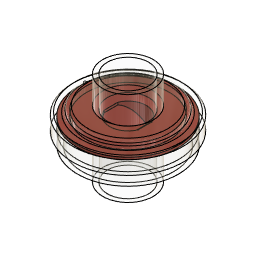
Patient Manifold v2 (Autodesk Fusion 360 design; units mm, degrees)
Autodesk Fusion 360 part; units mm, degrees
sketch "Sketch1" plane through (0, 0, 0) normal (0, 1, 0) x (1, 0, 0)
  line L0 (-20, 0) -> (-20, -10)
  line L1 (-20, -10) -> (-22, -10)
  line L2 (-22, -10) -> (-22, 0)
  line L3 (-22, 0) -> (-20, 0)
  line L4 (-11, -10.0136) -> (-11, 13.9248)
  line L5 (-11, 13.9248) -> (-9, 13.9248)
  line L6 (-9, 13.9248) -> (-9, -10.0136)
  line L7 (-9, -10.0136) -> (-11, -10.0136)
  line L8 (-20, -10) -> (-11, -10.0136)
  line L9 (-20, -8.4865) -> (-11, -8.4865)
  line L10 (-22, -5.5) -> (-24, -5.5)
  line L11 (-24, -5.5) -> (-24, -11.4635)
  line L12 (-23, -12.4635) -> (-20.5, -12.4635)
  line L13 (-22, -10) -> (-22, -11)
  line L14 (-22, -11) -> (-18, -11)
  line L15 (-18, -11) -> (-18, -13.5)
  line L16 (-18, -11) -> (0, -11)
  line L17 (0, -11) -> (0, -2.5)
  line L18 (0, -2.5) -> (-9, -10.0136)
  line L19 (-8.5, -11) -> (0, -4)
  line L20 (-18, -13.5) -> (-9, -13.5)
  line L21 (-9, -13.5) -> (-9, -26.8687)
  line L22 (-9, -26.8687) -> (-11, -26.8687)
  line L23 (-11, -26.8687) -> (-11, -15)
  line L24 (-11, -15) -> (-17.5, -15)
  line L25 (-9, -10.0136) -> (-9, -11)
  line L26 (0, -2.5) -> (-9, -2.5)
  arc A0 (-24, -11.4635) -> (-23, -12.4635) centre (-23, -11.4635) ccw
  arc A1 (-19.5, -13.4635) -> (-20.5, -12.4635) centre (-20.5, -13.4635) ccw
  spline S0 degree 5 poles (-19.5, -13.4635) (-19.5, -13.634) (-19.4835, -13.9431) (-19.4093, -14.312) (-19.2195, -14.6402) (-18.8414, -14.8679) (-18.4111, -14.9593) (-17.9961, -14.9926) (-17.6731, -15) (-17.5, -15) knots 0 0 0 0 0 0 0.2 0.4 0.6 0.8 1 1 1 1 1 1
  line L27 (-17.9, -15) -> (-17.1, -15)
  line L28 (-19.5, -13.1) -> (-19.5, -13.8271)
  dimension "d1" = 2
  dimension "d2" = 2
  dimension "d3" = 11
  dimension "d4" = 20
  dimension "d5" = 9
  dimension "d6" = 11
  dimension "d14" = 1
  constraint vertical L0
  constraint perpendicular L0 L1
  constraint perpendicular L1 L2
  constraint perpendicular L2 L3
  constraint perpendicular L3 L4
  constraint perpendicular L4 L5
  constraint perpendicular L5 L6
  constraint perpendicular L4 L7
  constraint coincident L0 L9.start
  constraint coincident L4 L9.end
  constraint perpendicular L4 L9
  constraint horizontal L10
  constraint perpendicular L10 L11
  constraint perpendicular L11 L12
  constraint perpendicular L1 L13
  constraint perpendicular L13 L14
  constraint perpendicular L14 L15
  constraint perpendicular L15 L16
  constraint perpendicular L14 L17
  constraint coincident L16 L19.start
  constraint coincident L17 L19.end
  constraint perpendicular L15 L20
  constraint perpendicular L20 L21
  constraint perpendicular L21 L22
  constraint perpendicular L20 L23
  constraint perpendicular L21 L24
  constraint midpoint L16 L25.end
  constraint coincident L6 L26.end
  constraint perpendicular L6 L26
  constraint tangent L12 A0
  constraint tangent L11 A0
  constraint tangent L12 A1
  constraint equal A0 A1
  constraint midpoint L24.end L27
  constraint coincident L24 L27.end
  constraint midpoint A1.start L28
  constraint tangent A1 L28
  measures "d1" distance of L4 L6
  measures "d2" distance of L0 L2 L3.end
  measures "d3" distance of origin L4
  measures "d4" distance of origin L0
  measures "d5" distance of L21 origin
  measures "d6" distance of L23 origin
  measures "d14" radius of A0
revolve "Revolve1" add sketch "Sketch1" angle 360 about axis through (0, 0, 1.75) along (0, 0, 1) contours L6 L18 L26 | L16 L17 L18 L19 L25 | L16 L17 L19 makes body 1
extrude "Extrude1" cut sketch "Sketch1" along normal through all and the other way through all contours L6 L18 L26 bodies 1
mirror "Mirror1" about plane through (0, 0, 0) normal (1, 0, 0) of "Extrude1"
shell "Shell1" thickness 1 removed faces 0 bodies 1
extrude "Extrude2" cut 1 faces at (-3.2811, 1.8539, 10) along direction (0, 0, 1) through all on bodies 1 bodies 1
revolve "Revolve2" add sketch "Sketch1" angle 360 about axis through (0, 0, 1.75) along (0, 0, 1) contours L1 L7 L8 L13 L14 L16 L25 bodies 1
revolve "Revolve3" add sketch "Sketch1" angle 360 about axis through (0, 0, 1.75) along (0, 0, 1) separate body contours L2 L10 L11 L12 L13 L14 L15 L20 L21 L22 L23 L24 A0 A1 S0 L27 makes body 2
revolve "Revolve4" add sketch "Sketch1" angle 360 about axis through (0, 0, 1.75) along (0, 0, 1) separate body contours L0 L1 L2 L3 | L0 L4 L8 L9 | L4 L5 L6 L7 makes body 3
revolve "Revolve5" cut sketch "Sketch1" angle 20 about axis through (0, 0, 1.75) along (0, 0, -1) contours L0 L4 L8 L9 bodies 3
pattern_circular "C-Pattern1" count 12 over 360 about axis through (0, 0, 1.75) along (0, 0, 1) of "Revolve5"
copy_body "Body->Comp1" bodies 1 removing the originals makes body 4 in component "Diaphragm"
copy_body "Body->Comp2" bodies 2 removing the originals makes body 5 in component "Top"
copy_body "Body->Comp3" bodies 3 removing the originals makes body 6 in component "Bottom"
component "Diaphragm" placed x (1, 0, 0) y (0, 1, 0) z (0, 0, 1) at (0, 0, 0)
component "Top" placed x (1, 0, 0) y (0, 1, 0) z (0, 0, 1) at (0, 0, 0)
component "Bottom" placed x (1, 0, 0) y (0, 1, 0) z (0, 0, 1) at (0, 0, 0)
named bodies: "Diaphragm", "Top", "Bottom"
